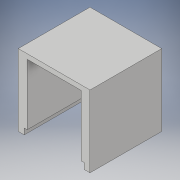
# Autodesk Inventor part: main body
Saved by Autodesk Inventor 2019.4 (Build 234330000, 330)
## iProperties
Created: 2020-11-09
Part Number: main body
Material: Generic
Document SubType Name: Modeling
Designer: caleb
Density: 1 g/cm^3
Appearance: Default
Author: caleb
Autodesk Inventor part; units mm, degrees
ref_plane "YZ Plane" through (0, 0, 0) normal (1, 0, 0) x (0, 1, 0)
ref_plane "XZ Plane" through (0, 0, 0) normal (0, 1, 0) x (-1, 0, 0)
ref_plane "XY Plane" through (0, 0, 0) normal (0, 0, 1) x (1, 0, 0)
sketch "Sketch1" plane through (0, 0, 0) normal (0, 1, 0) x (-1, 0, 0)
  line L0 (38.1, 38.1) -> (-38.1, 38.1)
  line L1 (-38.1, 38.1) -> (-38.1, -38.1)
  line L2 (-38.1, -38.1) -> (38.1, -38.1)
  line L3 (38.1, -38.1) -> (38.1, 38.1)
  point P0 (0, 0)
  dimension "d0" = 76.2
  dimension "d1" = 38.1
  dimension "d2" = 38.1
  constraints: 8 end point, 2 parallel, 2 perpendicular, 1 horizontal
  measures "d0" distance of L2.end L0.start
  measures "d1" distance from line of point (0, 0) L3
  measures "d2" distance from line of point (0, 0) L0
extrude "Extrusion1" add sketch "Sketch1" along normal blind 76.2
sketch "Sketch2" plane through (0, 0, 0) normal (0, -1, 0) x (1, 0, 0)
  line L0 (-38.1, 38.1) -> (38.1, 38.1) projected
  line L1 (38.1, -38.1) -> (-38.1, -38.1) projected
  line L2 (-28.575, 38.1) -> (28.575, 38.1)
  line L3 (28.575, 38.1) -> (28.575, -38.1)
  line L4 (28.575, -38.1) -> (-28.575, -38.1)
  line L5 (-28.575, -38.1) -> (-28.575, 38.1)
  point P0 (0, 0)
  dimension "d5" = 28.575
  dimension "d17" = 28.575
  constraints: 8 end point, 2 parallel, 2 point on line, 1 horizontal, 1 perpendicular
  measures "d5" distance from line of L5 point (0, 0)
  measures "d17" distance from line of L3 point (0, 0)
extrude "Extrusion2" cut sketch "Sketch2" against normal blind 50.8
sketch "Sketch4" plane through (-38.1, 76.2, 38.1) normal (0, 0, 1) x (1, 0, 0)
  line L0 (76.2, -76.2) -> (0, -76.2) projected
  line L1 (9.525, -76.2) -> (6.35, -76.2)
  line L2 (6.35, -76.2) -> (6.35, -69.85)
  line L3 (6.35, -69.85) -> (9.525, -69.85)
  line L4 (9.525, -69.85) -> (9.525, -76.2)
  line L5 (66.675, -76.2) -> (66.675, -25.4) projected
  line L6 (66.675, -76.2) -> (69.85, -76.2)
  line L7 (69.85, -76.2) -> (69.85, -69.85)
  line L8 (69.85, -69.85) -> (66.675, -69.85)
  line L9 (66.675, -69.85) -> (66.675, -76.2)
  line L10 (0, -76.2) -> (0, 0) projected
  line L11 (76.2, -76.2) -> (76.2, 0) projected
  point P0 (38.1, -76.2)
  dimension "d11" = 6.35
  dimension "d14" = 6.35
  dimension "d21" = 6.35
  dimension "d22" = 6.35
  constraints: 16 end point, 4 parallel, 2 horizontal, 2 perpendicular
  measures "d11" distance of L1.end L2.end
  measures "d14" distance of L6.end L7.end
  measures "d21" distance from line of L10 L2.end
  measures "d22" distance from line of L11 L7.end
extrude "Extrusion3" cut sketch "Sketch4" against normal blind 152.4
chamfer "Chamfer2" distance 20.32 angle 45 1 edges at (0, 50.8, 38.1) measured on face at (0, 50.8, 37.6)
body "Solid1"
